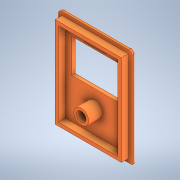
# Autodesk Inventor part: Enclosure v2
Saved by Autodesk Inventor 2022 (Build 260153000, 153)
## iProperties
Created: 2022-01-11
Part Number: Enclosure v2
Material: PLA Plastic
Document SubType Name: Modeling
Designer: chad
Density: 0.25 g/cm^3
Appearance: Generic(1)
Author: chad
Autodesk Inventor part; units mm, degrees
ref_plane "YZ Plane" through (0, 0, 0) normal (1, 0, 0) x (0, 1, 0)
ref_plane "XZ Plane" through (0, 0, 0) normal (0, 1, 0) x (-1, 0, 0)
ref_plane "XY Plane" through (0, 0, 0) normal (0, 0, 1) x (1, 0, 0)
sketch "Sketch2" plane through (0, 0, 0) normal (0, 0, 1) x (1, 0, 0)
  line L0 (0, 0) -> (42.2, 0)
  line L1 (42.2, 0) -> (42.2, 56.2)
  line L2 (42.2, 56.2) -> (0, 56.2)
  line L3 (0, 56.2) -> (0, 0)
  dimension "d0" = 42.2
  dimension "d1" = 56.2
  constraints: 8 end point, 2 parallel, 1 horizontal, 1 perpendicular
  measures "d0" distance of L2.end L1.end
  measures "d1" distance of L1.end L0.end
extrude "Extrusion1" add sketch "Sketch2" along normal blind 2
sketch "Sketch4" plane through (0, 0, 2) normal (0, 0, 1) x (1, 0, 0)
  line L0 (2.1, 2.1) -> (40.1, 2.1)
  line L1 (40.1, 2.1) -> (40.1, 54.1)
  line L2 (40.1, 54.1) -> (2.1, 54.1)
  line L3 (2.1, 54.1) -> (2.1, 2.1)
  line L4 (42.2, 0) -> (42.2, 56.2) projected
  line L5 (0, 56.2) -> (0, 0) projected
  line L6 (0, 0) -> (42.2, 0) projected
  line L7 (42.2, 56.2) -> (0, 56.2) projected
  dimension "d12" = 38
  dimension "d13" = 52
  dimension "d49" = 42.2
  dimension "d50" = 56.2
  dimension "d51" = 2.1
  dimension "d52" = 2.1
  constraints: 8 end point, 2 parallel, 1 horizontal, 1 perpendicular
  measures "d12" distance of L2.end L1.end
  measures "d13" distance of L1.end L0.end
  measures "d49" distance between parallel lines of L4 L5
  measures "d50" distance between parallel lines of L6 L7
  measures "d51" distance between parallel lines of L3 L5
  measures "d52" distance between parallel lines of L6 L0
extrude "Extrusion2" add sketch "Sketch4" along normal blind 4 contours L3 L2 L1 L0
sketch "Sketch5" plane through (0, 0, 6) normal (0, 0, 1) x (1, 0, 0)
  line L0 (4.1, 4.1) -> (38.1, 4.1)
  line L1 (38.1, 4.1) -> (38.1, 52.1)
  line L2 (38.1, 52.1) -> (4.1, 52.1)
  line L3 (4.1, 52.1) -> (4.1, 4.1)
  line L4 (40.1, 2.1) -> (40.1, 54.1) projected
  line L5 (2.1, 54.1) -> (2.1, 2.1) projected
  line L6 (2.1, 2.1) -> (40.1, 2.1) projected
  line L7 (40.1, 54.1) -> (2.1, 54.1) projected
  point P0 (0, 0)
  dimension "d16" = 34
  dimension "d17" = 48
  dimension "d45" = 38
  dimension "d46" = 2
  dimension "d47" = 52
  dimension "d48" = 2
  constraints: 8 end point, 2 parallel, 1 horizontal, 1 perpendicular
  measures "d16" distance of L2.end L1.end
  measures "d17" distance of L1.end L0.end
  measures "d45" distance between parallel lines of L4 L5
  measures "d46" distance between parallel lines of L3 L5
  measures "d47" distance between parallel lines of L6 L7
  measures "d48" distance between parallel lines of L0 L6
extrude "Extrusion3" cut sketch "Sketch5" against normal blind 4 contours L3 L2 L1 L0
sketch "Sketch6" plane through (0, 0, 2) normal (0, 0, 1) x (1, 0, 0)
  line L0 (7.6, 27.1) -> (34.6, 27.1)
  line L1 (34.6, 27.1) -> (34.6, 46.6)
  line L2 (34.6, 46.6) -> (7.6, 46.6)
  line L3 (7.6, 46.6) -> (7.6, 27.1)
  line L4 (15.1, 50.6) -> (27.1, 50.6)
  line L5 (27.1, 50.6) -> (27.1, 47.6)
  line L6 (27.1, 47.6) -> (15.1, 47.6)
  line L7 (15.1, 47.6) -> (15.1, 50.6)
  line L8 (4.1, 52.1) -> (38.1, 52.1) projected
  line L9 (38.1, 52.1) -> (38.1, 4.1) projected
  line L10 (4.1, 4.1) -> (4.1, 52.1) projected
  point P0 (0, 0)
  dimension "d20" = 27
  dimension "d21" = 19.5
  dimension "d22" = 12
  dimension "d23" = 3
  dimension "d24" = 1
  dimension "d25" = 1.5
  dimension "d42" = 34
  dimension "d43" = 3.5
  dimension "d44" = 11
  constraints: 16 end point, 4 parallel, 2 horizontal, 2 perpendicular
  measures "d20" distance of L2.end L1.end
  measures "d21" distance of L1.end L0.end
  measures "d22" distance of L5.end L6.end
  measures "d23" distance of L4.end L5.end
  measures "d24" distance between parallel lines of L2 L6
  measures "d25" distance between parallel lines of L4 L8
  measures "d42" distance between parallel lines of L9 L10
  measures "d43" distance between parallel lines of L3 L10
  measures "d44" distance between parallel lines of L10 L7
extrude "Extrusion4" cut sketch "Sketch6" against normal blind 1 contours L4 L5 L6 L7
extrude "Extrusion5" cut sketch "Sketch6" against normal blind 2 contours L3 L2 L1 L0
sketch "Sketch7" plane through (0, 0, 2) normal (0, 0, 1) x (1, 0, 0)
  circle A0 centre (21.1, 17.35) radius 2.75
  circle A1 centre (21.1, 17.35) radius 4.25
  line L0 (38.1, 4.1) -> (4.1, 4.1) projected
  line L1 (34.6, 27.1) -> (7.6, 27.1) projected
  line L2 (38.1, 52.1) -> (38.1, 4.1) projected
  line L3 (4.1, 4.1) -> (4.1, 52.1) projected
  point P0 (0, 0)
  dimension "d30" = 5.5
  dimension "d31" = 8.5
  dimension "d32" = 9
  dimension "d37" = 5.5
  dimension "d39" = 34
  dimension "d40" = 17
  constraints: 2 centre point, 1 coincident
  measures "d30" diameter of A0
  measures "d31" diameter of A1
  measures "d32" distance edge to line of A1 L0
  measures "d37" distance edge to line of A1 L1
  measures "d39" distance between parallel lines of L2 L3
  measures "d40" distance from line of L3 A1.centre
extrude "Extrusion6" add sketch "Sketch7" along normal blind 8
extrude "Extrusion7" cut sketch "Sketch7" against normal blind 1.75 contours A0
fillet "Fillet2" radius 1 3 edges at (21.1, 56.2, 0) (42.2, 28.1, 0) (0, 28.1, 0)
fillet "Fillet3" radius 2 4 edges at (0, 56.2, 1.5) (0.2929, 55.9071, 0.2929) (42.2, 56.2, 1.5) (41.9071, 55.9071, 0.2929)
equation "\"d51\" = -0.5 * d12 + 0.5 * d49"
equation "\"d52\" = -0.5 * d13 + 0.5 * d50"
equation "\"d46\" = -0.5 * d16 + 0.5 * d45"
equation "\"d48\" = -0.5 * d17 + 0.5 * d47"
equation "\"d43\" = -0.5 * d20 + 0.5 * d42"
equation "\"d44\" = -0.5 * d22 + 0.5 * d42"
equation "\"d40\" = 0.5 * d39"
body "Solid1"
